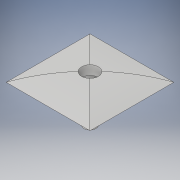
# Autodesk Inventor part: thumper-bumper-trigger-v2
Saved by Autodesk Inventor 2017 (Build 210142000, 142)
## iProperties
Created: 2017-02-22
Part Number: thumper-bumper-trigger-v2
Material: Generic
Document SubType Name: Modeling
Designer: John
Density: 1 g/cm^3
Appearance: Default
Author: John
Autodesk Inventor part; units mm, degrees
ref_plane "YZ Plane" through (0, 0, 0) normal (1, 0, 0) x (0, 1, 0)
ref_plane "XZ Plane" through (0, 0, 0) normal (0, 1, 0) x (-1, 0, 0)
ref_plane "XY Plane" through (0, 0, 0) normal (0, 0, 1) x (1, 0, 0)
sketch "Sketch1" plane through (0, 0, 0) normal (0, 1, 0) x (-1, 0, 0)
  line L0 (17.5, -17.5) -> (-17.5, -17.5)
  line L1 (-17.5, -17.5) -> (-17.5, 17.5)
  line L2 (-17.5, 17.5) -> (17.5, 17.5)
  line L3 (17.5, 17.5) -> (17.5, -17.5)
  line L4 (17.5, -17.5) -> (-17.5, 17.5) construction
  line L5 (-17.5, -17.5) -> (17.5, 17.5) construction
  point P0 (0, 0)
  dimension "d0" = 35
  dimension "d1" = 35
  constraints: 12 end point, 2 midpoint, 2 parallel, 1 horizontal, 1 perpendicular
  measures "d0" distance of L1.end L2.end
  measures "d1" distance of L0.end L1.end
extrude "Extrusion1" add sketch "Sketch1" along normal blind 4
sketch "Sketch3" plane through (17.5, 0, 17.5) normal (1, 0, 0) x (0, 0, -1)
  line L0 (35, 4) -> (0, 4) projected
  line L1 (0, 0) -> (35, 0) projected
  line L2 (0, 0) -> (35, 0)
  arc A0 (35, 0) -> (0, 0) centre (17.5, -36.2813) ccw
  point P0 (17.5, 4)
  constraints: 3 point on circle, 2 end point, 1 centre point, 1 horizontal, 1 midpoint
extrude "Extrusion3" cut sketch "Sketch3" against normal through all keep common part
sketch "Sketch4" plane through (17.5, 0, -17.5) normal (0, 0, -1) x (-1, 0, 0)
  line L0 (35, 0) -> (35, 4) projected
  line L1 (0, 0) -> (35, 0)
  line L2 (0, 0) -> (0, 4) projected
  line L3 (35, 0) -> (0, 0) projected
  arc A0 (35, 0) -> (0, 0) centre (17.5, -36.2812) ccw
  point P0 (17.5, 0)
  dimension "d31" = 4
  constraints: 2 end point, 2 point on circle, 1 centre point, 1 horizontal
  measures "d31" distance edge to line of A0 L1
extrude "Extrusion4" cut sketch "Sketch4" against normal through all keep common part
sketch "Sketch5" plane through (0, 0, 0) normal (0, -1, 0) x (1, 0, 0)
  circle A0 centre (0, 0) radius 3.5
  dimension "d14" = 7
  constraints: 1 centre point, 1 coincident
  measures "d14" diameter of A0
extrude "Extrusion5" cut sketch "Sketch5" against normal through all
sketch "Sketch6" plane through (0, 0, 0) normal (0, -1, 0) x (1, 0, 0)
  circle A0 centre (-6, -6) radius 2.5
  circle A1 centre (6, 6) radius 2.5
  circle A2 centre (6, -6) radius 2.5
  circle A3 centre (-6, 6) radius 2.5
  point P0 (0, 0)
  point P1 (0, 0)
  dimension "d17" = 5
  dimension "d18" = 5
  dimension "d19" = 6
  dimension "d20" = 6
  dimension "d21" = 6
  dimension "d22" = 6
  dimension "d25" = 5
  dimension "d26" = 5
  dimension "d27" = 6
  dimension "d28" = 6
  dimension "d29" = 6
  dimension "d30" = 6
  constraints: 4 centre point, 1 coincident
  measures "d17" diameter of A0
  measures "d18" diameter of A1
  measures "d19" horizontal distance of point (0, 0) A0.centre
  measures "d20" horizontal distance of A1.centre point (0, 0)
  measures "d21" horizontal distance of point (0, 0) A1.centre
  measures "d22" horizontal distance of point (0, 0) A0.centre
  measures "d25" diameter of A2
  measures "d26" diameter of A3
  measures "d27" horizontal distance of point (0, 0) A2.centre
  measures "d28" horizontal distance of point (0, 0) A2.centre
  measures "d29" horizontal distance of point (0, 0) A3.centre
  measures "d30" horizontal distance of point (0, 0) A3.centre
extrude "Extrusion6" add sketch "Sketch6" along normal blind 9.5 contours A0 | A1
sketch "Sketch7" plane through (0, 0, 0) normal (0, -1, 0) x (1, 0, 0)
  line L0 (-17.5, 17.5) -> (-17.5, -17.5) construction
  line L1 (-17.5, 0) -> (17.5, 0) construction
  line L2 (17.5, -17.5) -> (17.5, 17.5) construction
  circle A0 centre (0, 8.5) radius 2.5
  circle A1 centre (0, -8.5) radius 2.5
  line L3 (0, 0) -> (0, 8.5) construction
  dimension "d32" = 5
  dimension "d33" = 8.5
  constraints: 4 end point, 3 midpoint, 2 centre point, 1 symmetric about line, 1 vertical, 1 other
  measures "d32" diameter of A0
  measures "d33" distance of L3.start L3.end
extrude "Extrusion7" cut sketch "Sketch7" against normal blind 1.5
equation "\"d1\" = d0"
equation "\"d17\" = d18"
equation "\"d19\" = d21"
equation "\"d20\" = d27"
equation "\"d22\" = d27"
equation "\"d25\" = d18"
equation "\"d26\" = d18"
equation "\"d27\" = d21"
equation "\"d28\" = d21"
equation "\"d29\" = d21"
equation "\"d30\" = d21"
body "Solid1"
